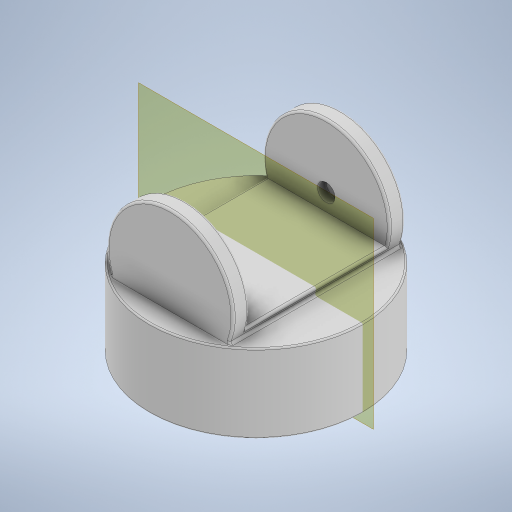
# Autodesk Inventor part: tutorial
Saved by Autodesk Inventor 2023 (Build 270158000, 158)
## iProperties
Created: 2023-03-30
Part Number: tutorial
Material: Ogólny
Document SubType Name: Modeling
Designer: Wiktor
Density: 1 g/cm^3
Appearance: Domyślna
Author: Wiktor
Autodesk Inventor part; units mm, degrees
ref_plane "XY Plane" through (0, 0, 0) normal (0, 0, 1) x (1, 0, 0)
sketch "Szkic1" plane through (0, 0, 0) normal (0, 0, 1) x (1, 0, 0)
  circle A0 centre (0, 0) radius 90
  dimension "d0" = 180
  constraints: 1 centre point, 1 coincident
  measures "d0" diameter of A0
extrude "Wyciągnięcie proste1" add sketch "Szkic1" along normal mid plane 245
ref_plane "Płaszczyzna konstrukcyjna1" through (0, -68, 0) normal (0, 1, 0) x (-1, 0, 0)
sketch "Szkic3" plane through (0, -68, 0) normal (0, 1, 0) x (-1, 0, 0)
  line L0 (-90, -122.5) -> (90, -122.5) projected
  circle A0 centre (0, 0) radius 152.0074
  constraints: 1 coincident, 3 other
extrude "Wyciągnięcie proste2" add sketch "Szkic3" along normal blind 32.75 and the other way blind 78.75
ref_plane "Płaszczyzna konstrukcyjna2" through (90, 0, 0) normal (1, 0, 0) x (0, 1, 0)
sketch "Szkic4" plane through (90, 0, 0) normal (1, 0, 0) x (0, 1, 0)
  line L0 (101.8163, 100.1343) -> (-24.1955, 100.1343)
  line L1 (-24.1955, 100.1343) -> (-24.1955, -100.1343)
  line L2 (-24.1955, -100.1343) -> (101.8163, -100.1343)
  line L3 (101.8163, -100.1343) -> (101.8163, 100.1343)
  line L4 (101.8163, 100.1343) -> (-24.1955, -100.1343) construction
  line L5 (-24.1955, 100.1343) -> (101.8163, -100.1343) construction
  point P0 (0, 0)
  constraints: 12 end point, 2 parallel, 1 horizontal, 1 perpendicular
extrude "Wyciągnięcie proste3" cut sketch "Szkic4" against normal blind 255.5
sketch "Szkic6" plane through (0, 0, -100.1343) normal (0, 0, 1) x (1, 0, 0)
  circle A0 centre (0, 0) radius 12.5
  dimension "d10" = 25
  constraints: 1 centre point, 1 coincident
  measures "d10" diameter of A0
extrude "Wyciągnięcie proste4" cut sketch "Szkic6" against normal blind 12.25
ref_plane "Płaszczyzna konstrukcyjna3" through (0, 0, 0) normal (0, 0, 1) x (1, 0, 0)
mirror "Odbij1" about plane through (0, 0, 0) normal (0, 0, 1) of "Wyciągnięcie proste4"
fillet "Zaokrąglenie1" radius 3 8 edges at (0, 90, 122.5) (0, 90, 100.1343) (-86.6867, -24.1955, 0) (0, 90, -100.1343) (0, 90, -122.5) (-82.8096, -35.25, 0) (82.8096, -35.25, 0) (86.6867, -24.1955, 0)
fillet "Zaokrąglenie2" radius 2 2 edges at (152.0074, -35.25, 0) (152.0074, -146.75, 0)
ref_plane "Płaszczyzna konstrukcyjna4" through (0, 0, 0) normal (0, 0, 1) x (1, 0, 0)
